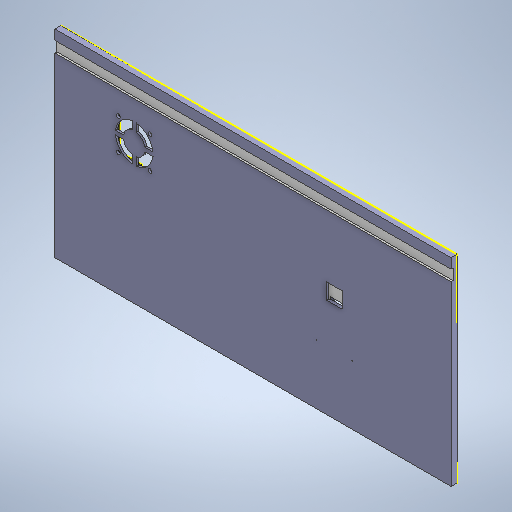
# Autodesk Inventor part: BackWall
Saved by Autodesk Inventor 2026.2 (Build 302298010, 298A)
## iProperties
Created: 2026-03-19
Part Number: BackWall
Material: Ogólny
Document SubType Name: Modeling
Designer: Patryk
Density: 1 g/cm^3
Appearance: Domyślna
Author: Patryk
Autodesk Inventor part; units mm, degrees
ref_plane "YZ Plane" through (0, 0, 0) normal (1, 0, 0) x (0, 1, 0)
ref_plane "XZ Plane" through (0, 0, 0) normal (0, 1, 0) x (-1, 0, 0)
ref_plane "XY Plane" through (0, 0, 0) normal (0, 0, 1) x (1, 0, 0)
sketch "Szkic1" plane through (0, 0, 0) normal (0, 0, 1) x (1, 0, 0)
  line L0 (200, 100) -> (-200, 100)
  line L1 (-200, 100) -> (-200, -100)
  line L2 (-200, -100) -> (200, -100)
  line L3 (200, -100) -> (200, 100)
  line L4 (200, 100) -> (-200, -100) construction
  line L5 (-200, 100) -> (200, -100) construction
  point P0 (0, 0)
  dimension "d0" = 400
  dimension "d1" = 200
  constraints: 12 end point, 2 midpoint, 2 parallel, 1 horizontal, 1 perpendicular
  measures "d0" distance of L2.end L1.end
  measures "d1" distance of L1.end L0.end
extrude "Wyciągnięcie proste1" add sketch "Szkic1" along normal mid plane 6
sketch "Szkic2" plane through (0, 0, 3) normal (0, 0, 1) x (1, 0, 0)
  circle A0 centre (-120, 40) radius 19
  line L0 (-200, 100) -> (-200, -100) projected
  line L1 (200, 100) -> (-200, 100) projected
  line L2 (-104, 24) -> (-136, 24)
  line L3 (-136, 24) -> (-136, 56)
  line L4 (-136, 56) -> (-104, 56)
  line L5 (-104, 56) -> (-104, 24)
  line L6 (-104, 24) -> (-136, 56) construction
  line L7 (-136, 24) -> (-104, 56) construction
  circle A1 centre (-136, 56) radius 2
  circle A2 centre (-104, 56) radius 2
  circle A3 centre (-104, 24) radius 2
  circle A4 centre (-136, 24) radius 2
  circle A5 centre (-120, 40) radius 11
  line L8 (-100, 20) -> (-140, 20)
  line L9 (-140, 20) -> (-140, 60)
  line L10 (-140, 60) -> (-100, 60)
  line L11 (-100, 60) -> (-100, 20)
  line L12 (-100, 20) -> (-140, 60) construction
  line L13 (-140, 20) -> (-100, 60) construction
  line L14 (-118, 20) -> (-122, 20)
  line L15 (-122, 20) -> (-122, 60)
  line L16 (-122, 60) -> (-118, 60)
  line L17 (-118, 60) -> (-118, 20)
  line L18 (-118, 20) -> (-122, 60) construction
  line L19 (-122, 20) -> (-118, 60) construction
  line L20 (-100, 38) -> (-140, 38)
  line L21 (-140, 38) -> (-140, 42)
  line L22 (-140, 42) -> (-100, 42)
  line L23 (-100, 42) -> (-100, 38)
  line L24 (-100, 38) -> (-140, 42) construction
  line L25 (-140, 38) -> (-100, 42) construction
  line L26 (100, -40) -> (64, -40)
  line L27 (-200, -100) -> (200, -100) projected
  circle A6 centre (64, -40) radius 0.5
  circle A7 centre (100, -40) radius 0.5
  line L28 (200, -100) -> (200, 100) projected
  line L29 (-200, 90) -> (200, 90)
  line L30 (200, 90) -> (200, 79)
  line L31 (200, 79) -> (-200, 79)
  line L32 (-200, 79) -> (-200, 90)
  point P0 (0, 0)
  point P1 (-122, 58.8944)
  point P2 (-138.8944, 42)
  point P3 (-130.8167, 42)
  point P4 (-122, 50.8167)
  point P5 (-101.1056, 42)
  point P6 (-118, 58.8944)
  point P7 (-118, 50.8167)
  point P8 (-109.1833, 42)
  point P9 (-118, 21.1056)
  point P10 (-101.1056, 38)
  point P11 (-109.1833, 38)
  point P12 (-118, 29.1833)
  point P13 (-130.8167, 38)
  point P14 (-138.8944, 38)
  point P15 (-122, 21.1056)
  point P16 (-122, 29.1833)
  dimension "d4" = 38
  dimension "d5" = 80
  dimension "d6" = 60
  dimension "d7" = 32
  dimension "d8" = 32
  dimension "d9" = 4
  dimension "d10" = 4
  dimension "d11" = 4
  dimension "d12" = 4
  dimension "d15" = 22
  dimension "d16" = 40
  dimension "d17" = 40
  dimension "d18" = 4
  dimension "d19" = 4
  dimension "d32" = 36
  dimension "d33" = 60
  dimension "d34" = 1
  dimension "d35" = 1
  dimension "d46" = 100
  dimension "d65" = 11
  dimension "d66" = 10
  constraints: 58 end point, 10 parallel, 8 centre point, 8 midpoint, 7 coincident, 6 horizontal, 5 perpendicular, 4 point on line
  measures "d4" diameter of A0
  measures "d5" distance from line of L0 A0.centre
  measures "d6" distance from line of L1 A0.centre
  measures "d7" distance of L3.end L4.end
  measures "d8" distance of L2.end L3.end
  measures "d9" diameter of A1
  measures "d10" diameter of A2
  measures "d11" diameter of A3
  measures "d12" diameter of A4
  measures "d15" diameter of A5
  measures "d16" distance of L9.end L10.end
  measures "d17" distance of L8.end L9.end
  measures "d18" distance of L15.end L16.end
  measures "d19" distance of L20.end L21.end
  measures "d32" distance of L26.start L26.end
  measures "d33" distance between parallel lines of L27 L26
  measures "d34" diameter of A6
  measures "d35" diameter of A7
  measures "d46" distance from line of L28 A7.centre
  measures "d65" distance between parallel lines of L29 L31
  measures "d66" distance between parallel lines of L29 L1
extrude "Wyciągnięcie proste3" cut sketch "Szkic2" against normal through all contours A2 L4 L5 | L5 L4 A2 | A3 L2 L5 | L5 L2 A3 | A1 L3 L4 | L4 L3 A1 | A4 L3 L2 | L2 L3 A4
extrude "Wyciągnięcie proste4" cut sketch "Szkic2" against normal through all contours L22 L5 A0 | A0 L5 L20 | L5 L22 A5 L17 L4 A0 | A0 L2 L17 A5 L20 L5 | L4 L17 A0 | A0 L17 L2 | L15 L4 A0 | L15 A5 L22 L3 A0 L4 | A0 L2 L15 | L2 A0 L3 L20 A5 L15 | L3 L22 A0 | A0 L20 L3
sketch "Szkic3" plane through (0, 0, -3) normal (0, 0, -1) x (-1, 0, 0)
  line L0 (118, 58.8944) -> (118, 50.8167) projected
  arc A0 (118, 50.8167) -> (109.1833, 42) centre (120, 40) ccw projected
  line L1 (109.1833, 42) -> (101.1056, 42) projected
  arc A1 (118, 58.8944) -> (101.1056, 42) centre (120, 40) ccw projected
  line L2 (101.1056, 38) -> (109.1833, 38) projected
  arc A2 (109.1833, 38) -> (118, 29.1833) centre (120, 40) ccw projected
  line L3 (118, 29.1833) -> (118, 21.1056) projected
  arc A3 (101.1056, 38) -> (118, 21.1056) centre (120, 40) ccw projected
  line L4 (138.8944, 42) -> (130.8167, 42) projected
  arc A4 (130.8167, 42) -> (122, 50.8167) centre (120, 40) ccw projected
  line L5 (122, 50.8167) -> (122, 58.8944) projected
  arc A5 (138.8944, 42) -> (122, 58.8944) centre (120, 40) ccw projected
  line L6 (122, 21.1056) -> (122, 29.1833) projected
  arc A6 (122, 29.1833) -> (130.8167, 38) centre (120, 40) ccw projected
  line L7 (130.8167, 38) -> (138.8944, 38) projected
  arc A7 (122, 21.1056) -> (138.8944, 38) centre (120, 40) ccw projected
  circle A8 centre (104, 24) radius 2 projected
  circle A9 centre (136, 24) radius 2 projected
  circle A10 centre (104, 56) radius 2 projected
  circle A11 centre (136, 56) radius 2 projected
  line L8 (200, -100) -> (200, 100) projected
  line L9 (200, 100) -> (-200, 100) projected
  line L10 (-200, 100) -> (-200, -100) projected
  line L11 (-200, -100) -> (200, -100) projected
  line L12 (140.5, 19.5) -> (99.5, 19.5)
  line L13 (99.5, 19.5) -> (99.5, 60.5)
  line L14 (99.5, 60.5) -> (140.5, 60.5)
  line L15 (140.5, 60.5) -> (140.5, 19.5)
  line L16 (140.5, 19.5) -> (99.5, 60.5) construction
  line L17 (99.5, 19.5) -> (140.5, 60.5) construction
  line L18 (200, -100) -> (-200, -100) projected
  line L19 (108, 19.5) -> (118, 19.5)
  line L20 (118, 19.5) -> (118, -100)
  line L21 (118, -100) -> (108, -100)
  line L22 (108, -100) -> (108, 19.5)
  point P0 (0, 0)
  dimension "d24" = 41
  dimension "d25" = 41
  dimension "d26" = 10
  dimension "d27" = 82
  constraints: 20 end point, 4 parallel, 2 horizontal, 2 midpoint, 2 perpendicular, 2 point on line
  measures "d24" distance of L13.end L14.end
  measures "d25" distance of L12.end L13.end
  measures "d26" distance between parallel lines of L22 L20
  measures "d27" distance between parallel lines of L8 L20
extrude "Wyciągnięcie proste5" cut sketch "Szkic3" against normal blind 3 contours L11 L22 L12 L20
extrude "Wyciągnięcie proste6" cut sketch "Szkic3" against normal blind 4 contours L0 A0 L1 A1 | L2 A2 L3 A3 | L4 A4 L5 A5 | L6 A6 L7 A7 | A8 | A9 | A10 | A11 | L12 L13 L14 L15
extrude "Wyciągnięcie proste7" cut sketch "Szkic2" against normal through all contours A6 | A7
sketch "Szkic4" plane through (0, 0, -3) normal (0, 0, -1) x (-1, 0, 0)
  circle A0 centre (-100, -40) radius 0.5 projected
  circle A1 centre (-64, -40) radius 0.5 projected
  line L0 (140.5, 19.5) -> (118, 19.5) projected
  line L1 (118, 19.5) -> (118, -100) projected
  line L2 (118, -100) -> (200, -100) projected
  line L3 (200, -100) -> (200, 100) projected
  line L4 (200, 100) -> (-200, 100) projected
  line L5 (-200, 100) -> (-200, -100) projected
  line L6 (-200, -100) -> (108, -100) projected
  line L7 (108, -100) -> (108, 19.5) projected
  line L8 (99.5, 19.5) -> (99.5, 60.5) projected
  line L9 (99.5, 60.5) -> (140.5, 60.5) projected
  line L10 (140.5, 60.5) -> (140.5, 19.5) projected
  line L11 (103.5, -100) -> (100.5, -100)
  line L12 (139.5, -100) -> (136.5, -100)
  line L13 (108, 19.5) -> (99.5, 19.5) projected
  point P0 (0, 0)
  constraints: 4 end point, 2 horizontal, 2 point on line
sketch "Szkic5" plane through (0, 0, 3) normal (0, 0, 1) x (1, 0, 0)
  circle A0 centre (100, -40) radius 0.5 projected
  circle A1 centre (64, -40) radius 0.5 projected
  line L0 (-118, 50.8167) -> (-118, 58.8944) projected
  arc A2 (-101.1056, 42) -> (-118, 58.8944) centre (-120, 40) ccw projected
  line L1 (-101.1056, 42) -> (-109.1833, 42) projected
  arc A3 (-109.1833, 42) -> (-118, 50.8167) centre (-120, 40) ccw projected
  line L2 (-109.1833, 38) -> (-101.1056, 38) projected
  arc A4 (-118, 21.1056) -> (-101.1056, 38) centre (-120, 40) ccw projected
  line L3 (-118, 21.1056) -> (-118, 29.1833) projected
  arc A5 (-118, 29.1833) -> (-109.1833, 38) centre (-120, 40) ccw projected
  line L4 (-130.8167, 42) -> (-138.8944, 42) projected
  arc A6 (-122, 58.8944) -> (-138.8944, 42) centre (-120, 40) ccw projected
  line L5 (-122, 58.8944) -> (-122, 50.8167) projected
  arc A7 (-122, 50.8167) -> (-130.8167, 42) centre (-120, 40) ccw projected
  line L6 (-122, 29.1833) -> (-122, 21.1056) projected
  arc A8 (-138.8944, 38) -> (-122, 21.1056) centre (-120, 40) ccw projected
  line L7 (-138.8944, 38) -> (-130.8167, 38) projected
  arc A9 (-130.8167, 38) -> (-122, 29.1833) centre (-120, 40) ccw projected
  circle A10 centre (-104, 24) radius 2 projected
  circle A11 centre (-136, 24) radius 2 projected
  circle A12 centre (-104, 56) radius 2 projected
  circle A13 centre (-136, 56) radius 2 projected
  line L8 (-200, 100) -> (-200, -100) projected
  line L9 (-200, -100) -> (200, -100) projected
  line L10 (200, -100) -> (200, 100) projected
  line L11 (200, 100) -> (-200, 100) projected
  line L12 (74, 16) -> (90, 16)
  line L13 (90, 16) -> (90, 0)
  line L14 (90, 0) -> (74, 0)
  line L15 (74, 0) -> (74, 16)
  line L16 (76, 16) -> (88, 16)
  line L17 (76, 0) -> (88, 0)
  line L18 (88, 0) -> (88, 3)
  line L19 (88, 3) -> (76, 3)
  line L20 (76, 3) -> (76, 0)
  point P0 (0, 0)
  dimension "d47" = 16
  dimension "d48" = 16
  dimension "d49" = 110
  dimension "d50" = 100
  dimension "d54" = 3
  dimension "d55" = 2
  dimension "d56" = 2
  constraints: 18 end point, 4 parallel, 3 horizontal, 2 perpendicular, 2 point on line
  measures "d47" distance of L13.end L14.end
  measures "d48" distance of L12.end L13.end
  measures "d49" distance between parallel lines of L10 L13
  measures "d50" distance between parallel lines of L9 L14
  measures "d54" distance of L18.end L17.end
  measures "d55" distance between parallel lines of L15 L20
  measures "d56" distance between parallel lines of L13 L18
extrude "Wyciągnięcie proste9" cut sketch "Szkic5" against normal through all contours L20 L19 L18 L14
extrude "Wyciągnięcie proste10" cut sketch "Szkic5" against normal blind 2 contours L12 L13 L14 L18 L19 L20 L15
sketch "Szkic6" plane through (0, 0, -3) normal (0, 0, -1) x (-1, 0, 0)
  line L0 (-76, 0) -> (-88, 0) projected
  line L1 (-88, 0) -> (-88, 3) projected
  line L2 (-88, 3) -> (-76, 3) projected
  line L3 (-76, 3) -> (-76, 0) projected
  circle A0 centre (-100, -40) radius 0.5 projected
  circle A1 centre (-64, -40) radius 0.5 projected
  line L4 (140.5, 19.5) -> (118, 19.5) projected
  line L5 (118, 19.5) -> (118, -100) projected
  line L6 (118, -100) -> (200, -100) projected
  line L7 (200, -100) -> (200, 100) projected
  line L8 (200, 100) -> (-200, 100) projected
  line L9 (-200, 100) -> (-200, -100) projected
  line L10 (-200, -100) -> (108, -100) projected
  line L11 (108, -100) -> (108, 19.5) projected
  line L12 (108, 19.5) -> (99.5, 19.5) projected
  line L13 (99.5, 19.5) -> (99.5, 60.5) projected
  line L14 (99.5, 60.5) -> (140.5, 60.5) projected
  line L15 (140.5, 60.5) -> (140.5, 19.5) projected
  line L16 (-90, 0) -> (-88, 0) projected
  line L17 (-88, 0) -> (-76, 0)
  line L18 (-76, 0) -> (-76, -100)
  line L19 (-76, -100) -> (-88, -100)
  line L20 (-88, -100) -> (-88, 0)
  line L21 (-100, -40) -> (-64, -40) construction
  line L22 (-100, -41) -> (-64, -41)
  line L23 (-64, -39) -> (-100, -39)
  arc A2 (-100, -39) -> (-100, -41) centre (-100, -40) ccw
  arc A3 (-64, -41) -> (-64, -39) centre (-64, -40) ccw
  point P0 (0, 0)
  point P1 (-82, -40)
  point P2 (-76, -39)
  point P3 (-88, -39)
  point P4 (-88, -41)
  point P5 (-76, -41)
  dimension "d61" = 12
  dimension "d62" = 2
  constraints: 16 end point, 4 point on circle, 4 tangent, 3 parallel, 2 centre point, 2 horizontal, 1 midpoint, 1 perpendicular, 1 point on line
  measures "d61" distance between parallel lines of L18 L20
  measures "d62" diameter of A3
extrude "Wyciągnięcie proste11" cut sketch "Szkic6" against normal blind 3 contours L18 L23 L20 L0 | L23 A3 L22 L18 | L18 L22 L20 L23 | L20 L22 A2 L23 | L18 L10 L20 L22 | A0 | A1
extrude "Wyciągnięcie proste12" cut sketch "Szkic2" against normal blind 2 contours L29 L28 L31 L0
